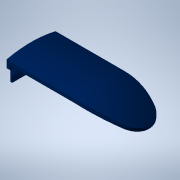
# Autodesk Inventor part: EGC-80-TB-KF_(AK)
Saved by Autodesk Inventor 2021 (Build 250183000, 183)
## iProperties
Created: 2026-04-25
Part Number: EGC-80-TB-KF_(AK)
Material: Generic
Catalog Web Link: www.3dfindit.com
Description: EGC-AK-TB-Abdekkappe
Vendor: FESTO
Document SubType Name: Modeling
Designer: psAdmin
Manufacturer: FESTO
Mass: 4.81888 g
Surface Area: 37.8015 cm^2
Volume: 4.81888 cm^3
Density: 1 g/cm^3
Appearance: PSOLRGB-0-145-219
Category: PARTsolutions
Company: FESTO
Title: EGC-80-TB-KF_(AK)
Author: Cadenas PARTsolutions
Comments: Abdekkappe
PSOL_IDENT_0: {$CADENAS_DATA/23d-libs/festo/parts/e/egc/parts/egc_tb_abdeckkappe.prj},177 {VTYP=3D},{NB=EGC-80-TB-
PSOL_IDENT_1: KF_(AK)},{LINA=EGC-80-TB-KF_(AK)},{NN=EGC-AK-TB},{DATE=12.11.2020 08:38:39},{GEOMDATE=27.06.2016 09:
PSOL_IDENT_2: 51:00},{VERSION=},{LINEID=30},{WBVAR=},{WBNUMERIC=}  {NB=EGC-80-TB-KF_(AK)},{LINA=EGC-80-TB-KF_(AK)}
PSOL_IDENT_3: ,{KT=DUMMY},{TYP=EGC-80-TB-KF},{VERS=3.000},{SIZE=80.000}
NB: EGC-80-TB-KF_(AK)
NN: EGC-AK-TB
NT: Abdekkappe
NBSYN: $TYP._(AK)
LINA: EGC-80-TB-KF_(AK)
CATALOG: Festo
TYP: EGC-80-TB-KF
VERS: 3
SIZE: 80
SUPPLIER: FESTO
ARTICLENO: EGC-80-TB-KF_(AK)
BOMINFO: EGC-80-TB-KF_(AK)
CREATOR: CADENAS GmbH
Autodesk Inventor part; units mm, degrees
sketch "Sketch_26" plane through (0, 0, 0) normal (0, 0, 1) x (1, 0, 0)
  line L0 (0, 15) -> (0, 0)
  line L1 (0, 0) -> (62.6, 0)
  line L2 (62.6, 0) -> (62.6, 15)
  line L3 (62.6, 15) -> (0, 15)
  constraints: 8 end point
extrude "Extrusion1" add sketch "Sketch_26" along normal mid plane 26
sketch "Sketch_1" plane through (0, 0, 0) normal (1, 0, 0) x (0, 0, -1)
  arc A0 (13, 11.25) -> (-13, 11.25) centre (0, -44.3333) ccw
  line L0 (13, 11.25) -> (13, 20.75)
  line L1 (13, 20.75) -> (-13, 20.75)
  line L2 (-13, 20.75) -> (-13, 11.25)
  constraints: 6 end point, 2 point on circle, 1 centre point
extrude "Extrusion2" cut sketch "Sketch_1" along normal blind 36.5
sketch "Sketch_12" plane through (0, 13.8, 0) normal (0, 1, 0) x (1, 0, 0)
  line L0 (-1, 16) -> (-1, -14)
  line L1 (-1, -14) -> (64, -14)
  line L2 (64, -14) -> (64, 16)
  line L3 (64, 16) -> (-1, 16)
  line L4 (0, 13) -> (0, -13)
  line L5 (0, -13) -> (36.5, -13)
  arc A0 (36.5, -13) -> (57.121, -8.5497) centre (36.5, 37) ccw
  arc A1 (57.121, -8.5497) -> (57.121, 8.5497) centre (53.2505, 0) ccw
  arc A2 (57.121, 8.5497) -> (36.5, 13) centre (36.5, -37) ccw
  line L6 (36.5, 13) -> (0, 13)
  constraints: 14 end point, 6 point on circle, 3 centre point
extrude "Extrusion3" cut sketch "Sketch_12" against normal blind 15
sketch "Sketch_3" plane through (36.5, 0, 0) normal (1, 0, 0) x (0, 0, -1)
  line L0 (13, -39.25) -> (-13, -39.25)
  arc A0 (13, 11.25) -> (-13, 11.25) centre (0, -44.3333) ccw
  line L1 (13, 11.25) -> (13, 25.75)
  line L2 (13, 25.75) -> (-13, 25.75)
  line L3 (-13, 25.75) -> (-13, 11.25)
  constraints: 8 end point, 2 point on circle, 1 centre point
revolve "Revolution1" cut sketch "Sketch_3" angle 35 about axis through (36.5, -39.25, -13) along (0, 0, -1)
sketch "Sketch_2" plane through (0, 0, 0) normal (0, 0, 1) x (1, 0, 0)
  line L0 (0, 7.3) -> (0, -51.7)
  line L1 (0, -51.7) -> (65, -51.7)
  line L2 (65, -51.7) -> (65, 3.3)
  arc A0 (65, 3.3) -> (36.5, 9.3) centre (32.036, -82.5916) ccw
  line L3 (36.5, 9.3) -> (2, 9.3)
  line L4 (2, 9.3) -> (2, 7.3)
  line L5 (2, 7.3) -> (0, 7.3)
  constraints: 12 end point, 2 point on circle, 1 centre point
extrude "Extrusion4" cut sketch "Sketch_2" along normal mid plane 26
sketch "Sketch_24" plane through (0, 0, 0) normal (0, 0, 1) x (1, 0, 0)
  line L0 (0, 10.75) -> (0, 0)
  line L1 (0, 0) -> (1, 0)
  line L2 (1, 0) -> (1, 3)
  line L3 (1, 3) -> (5.4745, 10.75)
  line L4 (5.4745, 10.75) -> (0, 10.75)
  constraints: 10 end point
extrude "Extrusion5" add sketch "Sketch_24" along normal mid plane 22
ref_plane "AK_XY" through (0, -0.05, 0) normal (-1, 0, 0) x (0, 0, -1)
ref_plane "AK_YZ" through (0, -0.05, 0) normal (0, 0, -1) x (0, -1, 0)
ref_plane "AK_ZX" through (0, -0.05, 0) normal (0, -1, 0) x (-1, 0, 0)
body "Solid1"
